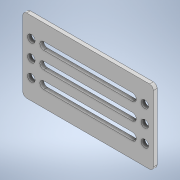
# Autodesk Inventor part: радиатор
Saved by Autodesk Inventor 2022 (Build 260153000, 153)
## iProperties
Created: 2022-07-09
Part Number: радиатор
Material: Типовые
Document SubType Name: Modeling
Designer: Константин
Density: 1 g/cm^3
Appearance: По умолчанию
Author: Константин
Autodesk Inventor part; units mm, degrees
ref_plane "YZ Plane" through (0, 0, 0) normal (1, 0, 0) x (0, 1, 0)
ref_plane "XZ Plane" through (0, 0, 0) normal (0, 1, 0) x (-1, 0, 0)
ref_plane "XY Plane" through (0, 0, 0) normal (0, 0, 1) x (1, 0, 0)
sketch "Эскиз1" plane through (0, 0, 0) normal (0, 0, 1) x (1, 0, 0)
  line L0 (-28.98, 25.9133) -> (40.02, 25.9133)
  line L1 (40.02, 25.9133) -> (40.02, -13.0867)
  line L2 (40.02, -13.0867) -> (-28.98, -13.0867)
  line L3 (-28.98, -13.0867) -> (-28.98, 25.9133)
  arc A0 (-17.98, 8.4133) -> (-17.98, 4.4133) centre (-17.98, 6.4133) ccw
  line L4 (-17.98, 8.4133) -> (5.52, 8.4133)
  line L5 (-17.98, 4.4133) -> (5.52, 4.4133)
  arc A1 (-17.98, 17.4133) -> (-17.98, 13.4133) centre (-17.98, 15.4133) ccw
  line L6 (-17.98, 17.4133) -> (5.52, 17.4133)
  line L7 (-17.98, 13.4133) -> (5.52, 13.4133)
  circle A2 centre (-24.48, 15.4133) radius 2
  circle A3 centre (-24.48, 6.4133) radius 2
  arc A4 (-17.98, -0.5867) -> (-17.98, -4.5867) centre (-17.98, -2.5867) ccw
  line L8 (-17.98, -4.5867) -> (5.52, -4.5867)
  line L9 (-17.98, -0.5867) -> (5.52, -0.5867)
  circle A5 centre (-24.48, -2.5867) radius 2
  arc A6 (29.02, 4.4133) -> (29.02, 8.4133) centre (29.02, 6.4133) ccw
  line L10 (29.02, 8.4133) -> (5.52, 8.4133)
  line L11 (29.02, 4.4133) -> (5.52, 4.4133)
  arc A7 (29.02, 13.4133) -> (29.02, 17.4133) centre (29.02, 15.4133) ccw
  line L12 (29.02, 17.4133) -> (5.52, 17.4133)
  line L13 (29.02, 13.4133) -> (5.52, 13.4133)
  circle A8 centre (35.52, 15.4133) radius 2
  circle A9 centre (35.52, 6.4133) radius 2
  circle A10 centre (35.52, -2.5867) radius 2
  line L14 (29.02, -4.5867) -> (5.52, -4.5867)
  arc A11 (29.02, -4.5867) -> (29.02, -0.5867) centre (29.02, -2.5867) ccw
  line L15 (29.02, -0.5867) -> (5.52, -0.5867)
  point P0 (0, 0)
  dimension "d0" = 69
  dimension "d1" = 39
  dimension "d3" = 4
  dimension "d8" = 4
  dimension "d9" = 4
  constraints: 32 end point, 12 centre point, 12 point on circle, 4 tangent, 3 horizontal, 2 perpendicular
  measures "d0" distance of L0.start L0.end
  measures "d1" distance of L2.end L0.start
  measures "d3" diameter of A0
  measures "d8" diameter of A2
  measures "d9" diameter of A3
extrude "Выдавливание1" add sketch "Эскиз1" along normal blind 2
fillet "Сопряжение1" radius 2 4 edges at (-28.98, 25.9133, 1) (40.02, 25.9133, 1) (40.02, -13.0867, 1) (-28.98, -13.0867, 1)
